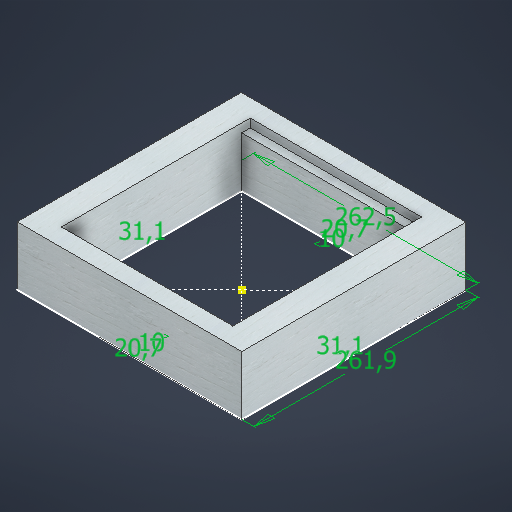
# Autodesk Inventor part: Melgueira-Sobreninho
Saved by Autodesk Inventor 2027 (Build 310192000, 192)
## iProperties
Created: 2026-10-01
Part Number: Melgueira-Sobreninho
Material: Genérico
Document SubType Name: Modeling
Designer: EspacoMaker
Density: 1 g/cm^3
Appearance: Padrão
Author: EspacoMaker
Autodesk Inventor part; units mm, degrees
ref_plane "YZ Plane" through (0, 0, 0) normal (1, 0, 0) x (0, 1, 0)
ref_plane "XZ Plane" through (0, 0, 0) normal (0, 1, 0) x (-1, 0, 0)
ref_plane "XY Plane" through (0, 0, 0) normal (0, 0, 1) x (1, 0, 0)
sketch "Esboço1" plane through (0, 0, 0) normal (0, 1, 0) x (-1, 0, 0)
  line L0 (131.25, 130.95) -> (-131.25, 130.95)
  line L1 (-131.25, 130.95) -> (-131.25, -130.95)
  line L2 (-131.25, -130.95) -> (131.25, -130.95)
  line L3 (131.25, -130.95) -> (131.25, 130.95)
  line L4 (131.25, 130.95) -> (-131.25, -130.95) construction
  line L5 (-131.25, 130.95) -> (131.25, -130.95) construction
  line L6 (-131.25, -110.25) -> (131.25, -110.25)
  line L7 (131.25, 110.25) -> (-131.25, 110.25)
  line L8 (100.15, -130.95) -> (100.15, 130.95)
  line L9 (-100.15, 130.95) -> (-100.15, -130.95)
  line L10 (131.25, 100.25) -> (-131.25, 100.25)
  line L11 (-131.25, -100.25) -> (131.25, -100.25)
  point P0 (0, 0)
  point P1 (-100.15, -100.25)
  point P2 (100.15, -100.25)
  point P3 (100.15, 100.25)
  point P4 (-100.15, 100.25)
  dimension "d0" = 262.5
  dimension "d1" = 261.9
  dimension "d2" = 20.7
  dimension "d3" = 20.7
  dimension "d4" = 31.1
  dimension "d5" = 31.1
  dimension "d6" = 10
  dimension "d7" = 10
  constraints: 24 end point, 8 parallel, 2 midpoint, 1 horizontal, 1 perpendicular
  measures "d0" distance of L2.end L1.end
  measures "d1" distance of L1.end L0.end
  measures "d2" distance between parallel lines of L2 L6
  measures "d3" distance between parallel lines of L0 L7
  measures "d4" distance between parallel lines of L3 L8
  measures "d5" distance between parallel lines of L1 L9
  measures "d6" distance between parallel lines of L7 L10
  measures "d7" distance between parallel lines of L6 L11
extrude "Extrusão1" add sketch "Esboço1" along normal blind 68.8
extrude "Extrusão2" cut sketch "Esboço1" along normal blind 68.8 contours L8 L11 L9 L10
sketch "Esboço2" plane through (0, 68.8, 0) normal (0, 1, 0) x (1, 0, 0)
  line L0 (100.15, 100.25) -> (-100.15, 100.25) projected
  line L1 (-100.15, -100.25) -> (-100.15, 100.25) projected
  line L2 (-100.15, 100.25) -> (-100.15, -100.25) projected
  line L3 (-100.15, 100.25) -> (-100.15, -100.25) projected
  line L4 (-100.15, -100.25) -> (-100.15, 100.25) projected
  line L5 (-131.25, 130.95) -> (-131.25, -130.95) projected
  line L6 (-131.25, 130.95) -> (-131.25, -130.95) projected
  line L7 (-131.25, 130.95) -> (-131.25, -130.95) projected
  line L8 (-131.25, 130.95) -> (-131.25, -130.95) projected
  line L9 (131.25, 130.95) -> (-131.25, 130.95) projected
  line L10 (-100.15, -100.25) -> (100.15, -100.25) projected
  line L11 (-131.25, -130.95) -> (131.25, -130.95) projected
  line L12 (100.15, 100.25) -> (-100.15, 100.25) projected
  line L13 (-100.15, 100.25) -> (-100.15, -100.25) projected
  line L14 (-100.15, -100.25) -> (100.15, -100.25) projected
  line L15 (100.15, -100.25) -> (100.15, 100.25) projected
  line L16 (-131.25, -130.95) -> (131.25, -130.95) projected
  line L17 (-131.25, 130.95) -> (-131.25, -130.95) projected
  line L18 (131.25, 130.95) -> (-131.25, 130.95) projected
  line L19 (131.25, -130.95) -> (131.25, 130.95) projected
  line L20 (131.25, -130.95) -> (131.25, 130.95) projected
  line L21 (100.15, -100.25) -> (100.15, 100.25) projected
  line L22 (-131.25, -130.95) -> (131.25, -130.95) projected
  line L23 (-131.25, -110.25) -> (131.25, -110.25) projected
  line L24 (-131.25, -100.25) -> (131.25, -100.25) projected
  line L25 (131.25, -130.95) -> (131.25, 130.95) projected
  line L26 (100.15, -130.95) -> (100.15, 130.95) projected
  line L27 (-100.15, 130.95) -> (-100.15, -130.95) projected
  line L28 (-131.25, -130.95) -> (131.25, 130.95) construction
  line L29 (-131.25, 130.95) -> (-131.25, -130.95) projected
  line L30 (131.25, -130.95) -> (-131.25, 130.95) construction
  line L31 (131.25, 100.25) -> (-131.25, 100.25) projected
  line L32 (131.25, 110.25) -> (-131.25, 110.25) projected
  line L33 (131.25, 130.95) -> (-131.25, 130.95) projected
  point P0 (0, 0)
  point P1 (0, 0)
  point P2 (-100.15, -110.25)
  point P3 (100.15, -110.25)
  point P4 (100.15, 110.25)
  point P5 (-100.15, 110.25)
  constraints: 6 other
extrude "Extrusão3" cut sketch "Esboço2" against normal blind 10 contours L0 L27 L32 L26 | L26 L23 L27 L10
